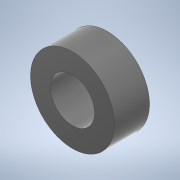
# Autodesk Inventor part: CC-0612-50B
Saved by Autodesk Inventor 2020.4 (Build 244396000, 396)
## iProperties
Created: 2021-09-06
Part Number: CC-0612-50B
Material: アセタール樹脂、黒
Document SubType Name: Modeling
Designer: Masato Kubotera
Density: 1.425 g/cm^3
Appearance: 滑らか - 黒
Mass: 0.291857 g
Surface Area: 3.07578 cm^2
Volume: 0.204812 cm^3
Description: 既製品
Author: Masato Kubotera
Comments: https://www.hirosugi-net.co.jp/shop/g/g31298/
Autodesk Inventor part; units mm, degrees
ref_plane "YZ Plane" through (0, 0, 0) normal (1, 0, 0) x (0, 1, 0)
ref_plane "XZ Plane" through (0, 0, 0) normal (0, 1, 0) x (-1, 0, 0)
ref_plane "XY Plane" through (0, 0, 0) normal (0, 0, 1) x (1, 0, 0)
sketch "スケッチ1" plane through (0, 0, 0) normal (0, 0, 1) x (1, 0, 0)
  circle A0 centre (0, 0) radius 3.15
  circle A1 centre (0, 0) radius 6
  dimension "d0" = 6.3
  dimension "d1" = 12
  constraints: 2 centre point, 2 coincident
  measures "d0" diameter of A0
  measures "d1" diameter of A1
extrude "押し出し1" add sketch "スケッチ1" along normal blind 5
